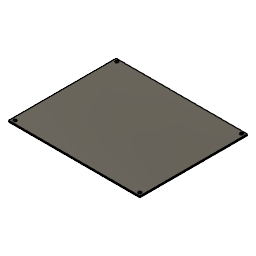
BB-BOT (Autodesk Fusion 360 archive; units mm, degrees)
design "Top plate"
Autodesk Fusion 360 part; units mm, degrees
sketch "Sketch1" plane through (0, 0, 45) normal (0, 0, 1) x (-1, 0, 0) in component "Top guard"
  arc A0 (130, -95) -> (130, -75) centre (130, -85) ccw
  line L0 (130, -75) -> (120, -75)
  line L1 (120, -75) -> (120, -35)
  line L2 (120, -35) -> (130, -35)
  arc A1 (130, -35) -> (130, -15) centre (130, -25) ccw
  line L3 (130, -15) -> (100, -15)
  line L4 (100, -15) -> (100, 50)
  line L5 (100, 50) -> (-100, 50)
  line L6 (-100, 50) -> (-100, -15)
  line L7 (-100, -15) -> (-130, -15)
  arc A2 (-130, -15) -> (-130, -35) centre (-130, -25) ccw
  line L8 (-130, -35) -> (-120, -35)
  line L9 (-120, -35) -> (-120, -75)
  line L10 (-120, -75) -> (-129.9999, -75)
  arc A3 (-129.9999, -75) -> (-129.9999, -95) centre (-129.9999, -85) ccw
  line L11 (-129.9999, -95) -> (-100, -95)
  line L12 (-100, -95) -> (-100, -160)
  line L13 (-100, -160) -> (-74, -160)
  line L14 (-74, -160) -> (-74, -115)
  line L15 (-74, -115) -> (74, -115)
  line L16 (74, -115) -> (74, -160)
  line L17 (74, -160) -> (100, -160)
  line L18 (100, -160) -> (100, -95)
  line L19 (100, -95) -> (130, -95)
  line L20 (83, 45) -> (83, -109)
  line L21 (-83, -109) -> (-83, 45)
  line L22 (-83, 45) -> (83, 45)
  circle A4 centre (130, -25) radius 4
  circle A5 centre (-129.9999, -85) radius 4
  circle A6 centre (-130, -25) radius 4
  circle A7 centre (130, -85) radius 4
  line L23 (100, -114) -> (-100, -114)
  line L24 (-100, -114) -> (-100, 50)
  line L25 (-100, 50) -> (100, 50)
  line L26 (100, 50) -> (100, -114)
  circle A8 centre (-95, -110) radius 2.25
  circle A9 centre (95, -110) radius 2.25
  circle A10 centre (95, 45) radius 2.25
  circle A11 centre (-95, 45) radius 2.25
  dimension "d7" = 4.5
  dimension "d8" = 4.5
  dimension "d9" = 4.5
  dimension "d10" = 4.5
  constraint horizontal L23
  constraint vertical L24
  constraint horizontal L25
  constraint vertical L26
  constraint coincident L5.end L6.start
  constraint coincident L18 L23.start
  measures "d7" diameter of A8
  measures "d8" diameter of A9
  measures "d9" diameter of A10
  measures "d10" diameter of A11
extrude "Extrude1" add sketch "Sketch1" along normal blind 2 contours L4 L5 L6 L12 L18 L23 L24 L25 L26 | A8 | A9 | A10 | A11 in component "Top guard"
extrude "Extrude2" cut sketch "Sketch1" along normal blind 2 contours A8 | A9 | A10 | A11 in component "Top guard"
component "Top guard" placed x (1, 0, 0) y (0, 1, 0) z (0, 0, 1) at (0, 0, 0)

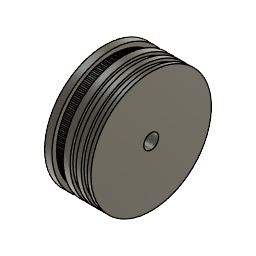
design "Wheel Hub"
Autodesk Fusion 360 part; units mm, degrees
sketch "Sketch1" plane through (0, 0, 0) normal (1, 0, 0) x (0, 1, 0) in component "Wheel-Hub"
  circle A0 centre (0, 0) radius 32.5
  dimension "d1" = 65
  constraint coincident A0.centre origin
  measures "d1" diameter of A0
extrude "Extrude1" add sketch "Sketch1" along normal blind 25 in component "Wheel-Hub"
sketch "Sketch2" plane through (25, 0, 0) normal (1, 0, 0) x (0, 1, 0) in component "Wheel-Hub"
  circle A0 centre (0, 0) radius 32.5
  circle A1 centre (0, 0) radius 4
  constraint coincident A0.centre A1.centre
extrude "Extrude2" cut sketch "Sketch2" against normal blind 25 contours A1 in component "Wheel-Hub"
sketch "Sketch3" plane through (25, 0, 0) normal (1, 0, 0) x (0, 1, 0) in component "Wheel-Hub"
  circle A0 centre (0, 0) radius 4
  circle A1 centre (0, 0) radius 32.5
  circle A2 centre (0, 0) radius 32.5
  circle A3 centre (0, 0) radius 31
  dimension "d6" = 65
  dimension "d7" = 62
  constraint coincident A0.centre A1.centre
  constraint concentric A2 A3
  measures "d6" diameter of A2
  measures "d7" diameter of A3
extrude "Extrude3" cut sketch "Sketch3" against normal blind 3.2 from surface at -2 contours A1 A2 in component "Wheel-Hub"
extrude "Extrude4" cut sketch "Sketch3" against normal blind 3.2 from surface at -8 contours A1 A2 in component "Wheel-Hub"
sketch "Sketch4" plane through (25, 0, 0) normal (1, 0, 0) x (0, 1, 0) in component "Wheel-Hub"
  circle A0 centre (0, 0) radius 4
  circle A1 centre (0, 0) radius 32.5
  circle A2 centre (0, 0) radius 32.5
  circle A3 centre (0, 0) radius 30
  dimension "d14" = 65
  dimension "d15" = 60
  constraint coincident A0.centre A1.centre
  measures "d14" diameter of A2
  measures "d15" diameter of A3
extrude "Extrude5" cut sketch "Sketch4" against normal blind 6 from surface at -15 contours A1 A2 in component "Wheel-Hub"
sketch "Sketch1 (2)" plane through (4, 0, 0) normal (1, 0, 0) x (0, 1, 0)
  circle A0 centre (0, 0) radius 30
  circle A1 centre (0, 0) radius 32.5
  line L0 (30, 0) -> (20.725, 0)
  line L1 (30, 0) -> (29.3, 0)
  line L2 (29.3, 0.5) -> (29.3, -0.5)
  line L3 (29.3, 0.5) -> (29.97, 0.7439)
  line L4 (29.3, -0.5) -> (29.97, -0.7439)
  arc A2 (29.97, -0.7439) -> (29.97, 0.7439) centre (20.7626, 0) ccw
  line L5 (29.3, 0) -> (29.315, 0)
  arc A3 (29.3, -0.5) -> (29.3, 0.5) centre (20.9742, 0) ccw
  line L6 (29.1677, 2.8263) -> (29.8162, 3.1226)
  arc A4 (29.9344, 1.6396) -> (29.8162, 3.1226) centre (20.697, 1.6496) ccw
  line L7 (29.2471, 1.8295) -> (29.9344, 1.6396)
  arc A5 (29.2471, 1.8295) -> (29.1677, 2.8263) centre (20.9079, 1.6664) ccw
  line L8 (28.8509, 5.1347) -> (29.4738, 5.4817)
  arc A6 (29.7095, 4.0127) -> (29.4738, 5.4817) centre (20.5005, 3.2888) ccw
  line L9 (29.0093, 4.1474) -> (29.7095, 4.0127)
  arc A7 (29.0093, 4.1474) -> (28.8509, 5.1347) centre (20.7094, 3.3223) ccw
  line L10 (28.3517, 7.4107) -> (28.9451, 7.806)
  arc A8 (29.2967, 6.3605) -> (28.9451, 7.806) centre (20.1744, 4.9071) ccw
  line L11 (28.5881, 6.4391) -> (29.2967, 6.3605)
  arc A9 (28.5881, 6.4391) -> (28.3517, 7.4107) centre (20.3799, 4.9571) ccw
  line L12 (27.6733, 9.6399) -> (28.2334, 10.081)
  arc A10 (28.6988, 8.668) -> (28.2334, 10.081) centre (19.7207, 6.4945) ccw
  line L13 (27.9861, 8.69) -> (28.6988, 8.668)
  arc A11 (27.9861, 8.69) -> (27.6733, 9.6399) centre (19.9217, 6.5606) ccw
  line L14 (26.82, 11.808) -> (27.3432, 12.2923)
  arc A12 (27.9194, 10.9207) -> (27.3432, 12.2923) centre (19.1424, 8.0408) ccw
  line L15 (27.2072, 10.8861) -> (27.9194, 10.9207)
  arc A13 (27.2072, 10.8861) -> (26.82, 11.808) centre (19.3375, 8.1227) ccw
  line L16 (25.797, 13.9016) -> (26.2802, 14.4259)
  arc A14 (26.9635, 13.1044) -> (26.2802, 14.4259) centre (18.4431, 9.5362) ccw
  line L17 (26.2563, 13.0133) -> (26.9635, 13.1044)
  arc A15 (26.2563, 13.0133) -> (25.797, 13.9016) centre (18.631, 9.6334) ccw
  line L18 (24.611, 15.9072) -> (25.051, 16.4683)
  arc A16 (25.8371, 15.2052) -> (25.051, 16.4683) centre (17.6271, 10.9714) ccw
  line L19 (25.1394, 15.0582) -> (25.8371, 15.2052)
  arc A17 (25.1394, 15.0582) -> (24.611, 15.9072) centre (17.8067, 11.0832) ccw
  line L20 (23.2694, 17.8122) -> (23.6634, 18.4065)
  arc A18 (24.5474, 17.2099) -> (23.6634, 18.4065) centre (16.6997, 12.3372) ccw
  line L21 (23.8636, 17.0079) -> (24.5474, 17.2099)
  arc A19 (23.8636, 17.0079) -> (23.2694, 17.8122) centre (16.8699, 12.4629) ccw
  line L22 (21.7806, 19.6047) -> (22.1262, 20.2284)
  arc A20 (23.1024, 19.1058) -> (22.1262, 20.2284) centre (15.6667, 13.625) ccw
  line L23 (22.4369, 18.8501) -> (23.1024, 19.1058)
  arc A21 (22.4369, 18.8501) -> (21.7806, 19.6047) centre (15.8264, 13.7638) ccw
  line L24 (20.1542, 21.2732) -> (20.4491, 21.9224)
  arc A22 (21.5115, 20.8809) -> (20.4491, 21.9224) centre (14.5347, 14.8266) ccw
  line L25 (20.8683, 20.5732) -> (21.5115, 20.8809)
  arc A23 (20.8683, 20.5732) -> (20.1542, 21.2732) centre (14.6828, 14.9777) ccw
  line L26 (18.4003, 22.8072) -> (18.6427, 23.4777)
  arc A24 (19.7845, 22.524) -> (18.6427, 23.4777) centre (13.3108, 15.9345) ccw
  line L27 (19.1678, 22.1661) -> (19.7845, 22.524)
  arc A25 (19.1678, 22.1661) -> (18.4003, 22.8072) centre (13.4464, 16.0969) ccw
  line L28 (16.5301, 24.197) -> (16.7184, 24.8847)
  arc A26 (17.9324, 24.0246) -> (16.7184, 24.8847) centre (12.0027, 16.9417) ccw
  line L29 (17.3461, 23.6189) -> (17.9324, 24.0246)
  arc A27 (17.3461, 23.6189) -> (16.5301, 24.197) centre (12.125, 17.1143) ccw
  line L30 (14.5554, 25.4338) -> (14.6885, 26.1343)
  arc A28 (15.9669, 25.3734) -> (14.6885, 26.1343) centre (10.6187, 17.8418) ccw
  line L31 (15.4147, 24.9224) -> (15.9669, 25.3734)
  arc A29 (15.4147, 24.9224) -> (14.5554, 25.4338) centre (10.7269, 18.0235) ccw
  line L32 (12.4887, 26.5099) -> (12.5657, 27.2187)
  arc A30 (13.9005, 26.5618) -> (12.5657, 27.2187) centre (9.1676, 18.629) ccw
  line L33 (13.3859, 26.0683) -> (13.9005, 26.5618)
  arc A31 (13.3859, 26.0683) -> (12.4887, 26.5099) centre (9.261, 18.8188) ccw
  line L34 (10.343, 27.4183) -> (10.3634, 28.131)
  arc A32 (11.7463, 27.5822) -> (10.3634, 28.131) centre (7.6586, 19.2985) ccw
  line L35 (11.2725, 27.0494) -> (11.7463, 27.5822)
  arc A33 (11.2725, 27.0494) -> (10.343, 27.4183) centre (7.7366, 19.4951) ccw
  line L36 (8.1319, 28.1534) -> (8.0957, 28.8655)
  arc A34 (9.5177, 28.4283) -> (8.0957, 28.8655) centre (6.1011, 19.846) ccw
  line L37 (9.0877, 27.8595) -> (9.5177, 28.4283)
  arc A35 (9.0877, 27.8595) -> (8.1319, 28.1534) centre (6.1633, 20.0482) ccw
  line L38 (5.8694, 28.7105) -> (5.7767, 29.4174)
  arc A36 (7.229, 29.0946) -> (5.7767, 29.4174) centre (4.505, 20.268) ccw
  line L39 (6.8456, 28.4935) -> (7.229, 29.0946)
  arc A37 (6.8456, 28.4935) -> (5.8694, 28.7105) centre (4.5509, 20.4745) ccw
  line L40 (3.5698, 29.086) -> (3.4212, 29.7834)
  arc A38 (4.8946, 29.577) -> (3.4212, 29.7834) centre (2.8805, 20.5618) ccw
  line L41 (4.5601, 28.9473) -> (4.8946, 29.577)
  arc A39 (4.5601, 28.9473) -> (3.5698, 29.086) centre (2.9099, 20.7713) ccw
  line L42 (1.2476, 29.2777) -> (1.0441, 29.961)
  arc A40 (2.5292, 29.8724) -> (1.0441, 29.961) centre (1.2378, 20.7257) ccw
  line L43 (2.2458, 29.2181) -> (2.5292, 29.8724)
  arc A41 (2.2458, 29.2181) -> (1.2476, 29.2777) centre (1.2504, 20.9369) ccw
  line L44 (-1.0824, 29.2843) -> (-1.3396, 29.9493)
  arc A42 (0.1478, 29.9789) -> (-1.3396, 29.9493) centre (-0.4128, 20.7585) ccw
  line L45 (-0.0826, 29.3041) -> (0.1478, 29.9789)
  arc A43 (-0.0826, 29.3041) -> (-1.0824, 29.2843) centre (-0.417, 20.97) ccw
  line L46 (-3.4057, 29.1057) -> (-3.7148, 29.7482)
  arc A44 (-2.2344, 29.8958) -> (-3.7148, 29.7482) centre (-2.0608, 20.6601) ccw
  line L47 (-2.4106, 29.2049) -> (-2.2344, 29.8958)
  arc A45 (-2.4106, 29.2049) -> (-3.4057, 29.1057) centre (-2.0818, 20.8706) ccw
  line L48 (-5.7074, 28.7431) -> (-6.0666, 29.359)
  arc A46 (-4.6026, 29.6238) -> (-6.0666, 29.359) centre (-3.6957, 20.431) ccw
  line L49 (-4.7233, 28.9211) -> (-4.6026, 29.6238)
  arc A47 (-4.7233, 28.9211) -> (-5.7074, 28.7431) centre (-3.7334, 20.6392) ccw
  line L50 (-7.973, 28.1988) -> (-8.38, 28.7842)
  arc A48 (-6.9417, 29.1645) -> (-8.38, 28.7842) centre (-5.3073, 20.0728) ccw
  line L51 (-7.0062, 28.4544) -> (-6.9417, 29.1645)
  arc A49 (-7.0062, 28.4544) -> (-7.973, 28.1988) centre (-5.3613, 20.2774) ccw
  line L52 (-10.1882, 27.4762) -> (-10.6404, 28.0274)
  arc A50 (-9.2369, 28.5208) -> (-10.6404, 28.0274) centre (-6.8853, 19.5877) ccw
  line L53 (-9.2447, 27.8078) -> (-9.2369, 28.5208)
  arc A51 (-9.2447, 27.8078) -> (-10.1882, 27.4762) centre (-6.9554, 19.7873) ccw
  line L54 (-12.3389, 26.5799) -> (-12.8335, 27.0934)
  arc A52 (-11.4736, 27.6967) -> (-12.8335, 27.0934) centre (-8.4198, 18.9788) ccw
  line L55 (-11.4248, 26.9854) -> (-11.4736, 27.6967)
  arc A53 (-11.4248, 26.9854) -> (-12.3389, 26.5799) centre (-8.5056, 19.1721) ccw
  line L56 (-14.4117, 25.5155) -> (-14.9456, 25.9882)
  arc A54 (-13.6379, 26.6976) -> (-14.9456, 25.9882) centre (-9.901, 18.2498) ccw
  line L57 (-13.5327, 25.9924) -> (-13.6379, 26.6976)
  arc A55 (-13.5327, 25.9924) -> (-14.4117, 25.5155) centre (-10.0019, 18.4358) ccw
  line L58 (-16.3934, 24.2899) -> (-16.9631, 24.7186)
  arc A56 (-15.7159, 25.5297) -> (-16.9631, 24.7186) centre (-11.3197, 17.4055) ccw
  line L59 (-15.5551, 24.8351) -> (-15.7159, 25.5297)
  arc A57 (-15.5551, 24.8351) -> (-16.3934, 24.2899) centre (-11.435, 17.5828) ccw
  line L60 (-18.2714, 22.9106) -> (-18.8733, 23.2927)
  arc A58 (-17.6946, 24.2003) -> (-18.8733, 23.2927) centre (-12.6667, 16.4511) ccw
  line L61 (-17.479, 23.5207) -> (-17.6946, 24.2003)
  arc A59 (-17.479, 23.5207) -> (-18.2714, 22.9106) centre (-12.7958, 16.6187) ccw
  line L62 (-20.0339, 21.3865) -> (-20.6643, 21.7196)
  arc A60 (-19.5613, 22.718) -> (-20.6643, 21.7196) centre (-13.9337, 15.3927) ccw
  line L63 (-19.2925, 22.0576) -> (-19.5613, 22.718)
  arc A61 (-19.2925, 22.0576) -> (-20.0339, 21.3865) centre (-14.0757, 15.5496) ccw
  line L64 (-21.6697, 19.7272) -> (-22.3246, 20.0092)
  arc A62 (-21.3045, 21.092) -> (-22.3246, 20.0092) centre (-15.1127, 14.237) ccw
  line L65 (-20.984, 20.4551) -> (-21.3045, 21.092)
  arc A63 (-20.984, 20.4551) -> (-21.6697, 19.7272) centre (-15.2666, 14.3821) ccw
  line L66 (-23.1685, 17.9432) -> (-23.8438, 18.1722)
  arc A64 (-22.9129, 19.3327) -> (-23.8438, 18.1722) centre (-16.196, 12.9913) ccw
  line L67 (-22.5428, 18.7233) -> (-22.9129, 19.3327)
  arc A65 (-22.5428, 18.7233) -> (-23.1685, 17.9432) centre (-16.361, 13.1237) ccw
  line L68 (-24.5209, 16.0458) -> (-25.2122, 16.2204)
  arc A66 (-24.3764, 17.4512) -> (-25.2122, 16.2204) centre (-17.177, 11.6635) ccw
  line L69 (-23.9591, 16.8731) -> (-24.3764, 17.4512)
  arc A67 (-23.9591, 16.8731) -> (-24.5209, 16.0458) centre (-17.352, 11.7823) ccw
  line L70 (-25.7182, 14.0468) -> (-26.4212, 14.166)
  arc A68 (-25.6859, 15.4593) -> (-26.4212, 14.166) centre (-18.0493, 10.2619) ccw
  line L71 (-25.224, 14.9162) -> (-25.6859, 15.4593)
  arc A69 (-25.224, 14.9162) -> (-25.7182, 14.0468) centre (-18.2333, 10.3665) ccw
  line L72 (-26.7529, 11.9591) -> (-27.4632, 12.022)
  arc A70 (-26.8329, 13.3697) -> (-27.4632, 12.022) centre (-18.8076, 8.7954) ccw
  line L73 (-26.3293, 12.865) -> (-26.8329, 13.3697)
  arc A71 (-26.3293, 12.865) -> (-26.7529, 11.9591) centre (-18.9992, 8.8851) ccw
  line L74 (-27.6185, 9.7958) -> (-28.3315, 9.8021)
  arc A72 (-27.8103, 11.1955) -> (-28.3315, 9.8021) centre (-19.4469, 7.2734) ccw
  line L75 (-27.2682, 10.7324) -> (-27.8103, 11.1955)
  arc A73 (-27.2682, 10.7324) -> (-27.6185, 9.7958) centre (-19.6451, 7.3475) ccw
  line L76 (-28.3095, 7.5705) -> (-29.0207, 7.5202)
  arc A74 (-28.6119, 8.9506) -> (-29.0207, 7.5202) centre (-19.9633, 5.7053) ccw
  line L77 (-28.0347, 8.532) -> (-28.6119, 8.9506)
  arc A75 (-28.0347, 8.532) -> (-28.3095, 7.5705) centre (-20.1668, 5.7634) ccw
  line L78 (-28.8215, 5.2974) -> (-29.5264, 5.1907)
  arc A76 (-29.2326, 6.6491) -> (-29.5264, 5.1907) centre (-20.3535, 4.1012) ccw
  line L79 (-28.6239, 6.2777) -> (-29.2326, 6.6491)
  arc A77 (-28.6239, 6.2777) -> (-28.8215, 5.2974) centre (-20.5609, 4.143) ccw
  line L80 (-29.1512, 2.9908) -> (-29.8455, 2.8284)
  arc A78 (-29.6684, 4.3055) -> (-29.8455, 2.8284) centre (-20.615, 2.4711) ccw
  line L81 (-29.0322, 3.9837) -> (-29.6684, 4.3055)
  arc A79 (-29.0322, 3.9837) -> (-29.1512, 2.9908) centre (-20.8251, 2.4963) ccw
  line L82 (-29.2967, 0.6653) -> (-29.9759, 0.4482)
  arc A80 (-29.9167, 1.9348) -> (-29.9759, 0.4482) centre (-20.7462, 0.8254) ccw
  line L83 (-29.257, 1.6645) -> (-29.9167, 1.9348)
  arc A81 (-29.257, 1.6645) -> (-29.2967, 0.6653) centre (-20.9576, 0.8339) ccw
  line L84 (-29.257, -1.6645) -> (-29.9167, -1.9348)
  arc A82 (-29.9759, -0.4482) -> (-29.9167, -1.9348) centre (-20.7462, -0.8254) ccw
  line L85 (-29.2967, -0.6653) -> (-29.9759, -0.4482)
  arc A83 (-29.2967, -0.6653) -> (-29.257, -1.6645) centre (-20.9576, -0.8339) ccw
  line L86 (-29.0322, -3.9837) -> (-29.6684, -4.3055)
  arc A84 (-29.8455, -2.8284) -> (-29.6684, -4.3055) centre (-20.615, -2.4711) ccw
  line L87 (-29.1512, -2.9908) -> (-29.8455, -2.8284)
  arc A85 (-29.1512, -2.9908) -> (-29.0322, -3.9837) centre (-20.8251, -2.4963) ccw
  line L88 (-28.6239, -6.2777) -> (-29.2326, -6.6491)
  arc A86 (-29.5264, -5.1907) -> (-29.2326, -6.6491) centre (-20.3535, -4.1012) ccw
  line L89 (-28.8215, -5.2974) -> (-29.5264, -5.1907)
  arc A87 (-28.8215, -5.2974) -> (-28.6239, -6.2777) centre (-20.5609, -4.143) ccw
  line L90 (-28.0347, -8.532) -> (-28.6119, -8.9506)
  arc A88 (-29.0207, -7.5202) -> (-28.6119, -8.9506) centre (-19.9633, -5.7053) ccw
  line L91 (-28.3095, -7.5705) -> (-29.0207, -7.5202)
  arc A89 (-28.3095, -7.5705) -> (-28.0347, -8.532) centre (-20.1668, -5.7634) ccw
  line L92 (-27.2682, -10.7324) -> (-27.8103, -11.1955)
  arc A90 (-28.3315, -9.8021) -> (-27.8103, -11.1955) centre (-19.4469, -7.2734) ccw
  line L93 (-27.6185, -9.7958) -> (-28.3315, -9.8021)
  arc A91 (-27.6185, -9.7958) -> (-27.2682, -10.7324) centre (-19.6451, -7.3475) ccw
  line L94 (-26.3293, -12.865) -> (-26.8329, -13.3697)
  arc A92 (-27.4632, -12.022) -> (-26.8329, -13.3697) centre (-18.8076, -8.7954) ccw
  line L95 (-26.7529, -11.9591) -> (-27.4632, -12.022)
  arc A93 (-26.7529, -11.9591) -> (-26.3293, -12.865) centre (-18.9992, -8.8851) ccw
  line L96 (-25.224, -14.9162) -> (-25.6859, -15.4593)
  arc A94 (-26.4212, -14.166) -> (-25.6859, -15.4593) centre (-18.0493, -10.2619) ccw
  line L97 (-25.7182, -14.0468) -> (-26.4212, -14.166)
  arc A95 (-25.7182, -14.0468) -> (-25.224, -14.9162) centre (-18.2333, -10.3665) ccw
  line L98 (-23.9591, -16.8731) -> (-24.3764, -17.4512)
  arc A96 (-25.2122, -16.2204) -> (-24.3764, -17.4512) centre (-17.177, -11.6635) ccw
  line L99 (-24.5209, -16.0458) -> (-25.2122, -16.2204)
  arc A97 (-24.5209, -16.0458) -> (-23.9591, -16.8731) centre (-17.352, -11.7823) ccw
  line L100 (-22.5428, -18.7233) -> (-22.9129, -19.3327)
  arc A98 (-23.8438, -18.1722) -> (-22.9129, -19.3327) centre (-16.196, -12.9913) ccw
  line L101 (-23.1685, -17.9432) -> (-23.8438, -18.1722)
  arc A99 (-23.1685, -17.9432) -> (-22.5428, -18.7233) centre (-16.361, -13.1237) ccw
  line L102 (-20.984, -20.4551) -> (-21.3045, -21.092)
  arc A100 (-22.3246, -20.0092) -> (-21.3045, -21.092) centre (-15.1127, -14.237) ccw
  line L103 (-21.6697, -19.7272) -> (-22.3246, -20.0092)
  arc A101 (-21.6697, -19.7272) -> (-20.984, -20.4551) centre (-15.2666, -14.3821) ccw
  line L104 (-19.2925, -22.0576) -> (-19.5613, -22.718)
  arc A102 (-20.6643, -21.7196) -> (-19.5613, -22.718) centre (-13.9337, -15.3927) ccw
  line L105 (-20.0339, -21.3865) -> (-20.6643, -21.7196)
  arc A103 (-20.0339, -21.3865) -> (-19.2925, -22.0576) centre (-14.0757, -15.5496) ccw
  line L106 (-17.479, -23.5207) -> (-17.6946, -24.2003)
  arc A104 (-18.8733, -23.2927) -> (-17.6946, -24.2003) centre (-12.6667, -16.4511) ccw
  line L107 (-18.2714, -22.9106) -> (-18.8733, -23.2927)
  arc A105 (-18.2714, -22.9106) -> (-17.479, -23.5207) centre (-12.7958, -16.6187) ccw
  line L108 (-15.5551, -24.8351) -> (-15.7159, -25.5297)
  arc A106 (-16.9631, -24.7186) -> (-15.7159, -25.5297) centre (-11.3197, -17.4055) ccw
  line L109 (-16.3934, -24.2899) -> (-16.9631, -24.7186)
  arc A107 (-16.3934, -24.2899) -> (-15.5551, -24.8351) centre (-11.435, -17.5828) ccw
  line L110 (-13.5327, -25.9924) -> (-13.6379, -26.6976)
  arc A108 (-14.9456, -25.9882) -> (-13.6379, -26.6976) centre (-9.901, -18.2498) ccw
  line L111 (-14.4117, -25.5155) -> (-14.9456, -25.9882)
  arc A109 (-14.4117, -25.5155) -> (-13.5327, -25.9924) centre (-10.0019, -18.4358) ccw
  line L112 (-11.4248, -26.9854) -> (-11.4736, -27.6967)
  arc A110 (-12.8335, -27.0934) -> (-11.4736, -27.6967) centre (-8.4198, -18.9788) ccw
  line L113 (-12.3389, -26.5799) -> (-12.8335, -27.0934)
  arc A111 (-12.3389, -26.5799) -> (-11.4248, -26.9854) centre (-8.5056, -19.1721) ccw
  line L114 (-9.2447, -27.8078) -> (-9.2369, -28.5208)
  arc A112 (-10.6404, -28.0274) -> (-9.2369, -28.5208) centre (-6.8853, -19.5877) ccw
  line L115 (-10.1882, -27.4762) -> (-10.6404, -28.0274)
  arc A113 (-10.1882, -27.4762) -> (-9.2447, -27.8078) centre (-6.9554, -19.7873) ccw
  line L116 (-7.0062, -28.4544) -> (-6.9417, -29.1645)
  arc A114 (-8.38, -28.7842) -> (-6.9417, -29.1645) centre (-5.3073, -20.0728) ccw
  line L117 (-7.973, -28.1988) -> (-8.38, -28.7842)
  arc A115 (-7.973, -28.1988) -> (-7.0062, -28.4544) centre (-5.3613, -20.2774) ccw
  line L118 (-4.7233, -28.9211) -> (-4.6026, -29.6238)
  arc A116 (-6.0666, -29.359) -> (-4.6026, -29.6238) centre (-3.6957, -20.431) ccw
  line L119 (-5.7074, -28.7431) -> (-6.0666, -29.359)
  arc A117 (-5.7074, -28.7431) -> (-4.7233, -28.9211) centre (-3.7334, -20.6392) ccw
  line L120 (-2.4106, -29.2049) -> (-2.2344, -29.8958)
  arc A118 (-3.7148, -29.7482) -> (-2.2344, -29.8958) centre (-2.0608, -20.6601) ccw
  line L121 (-3.4057, -29.1057) -> (-3.7148, -29.7482)
  arc A119 (-3.4057, -29.1057) -> (-2.4106, -29.2049) centre (-2.0818, -20.8706) ccw
  line L122 (-0.0826, -29.3041) -> (0.1478, -29.9789)
  arc A120 (-1.3396, -29.9493) -> (0.1478, -29.9789) centre (-0.4128, -20.7585) ccw
  line L123 (-1.0824, -29.2843) -> (-1.3396, -29.9493)
  arc A121 (-1.0824, -29.2843) -> (-0.0826, -29.3041) centre (-0.417, -20.97) ccw
  line L124 (2.2458, -29.2181) -> (2.5292, -29.8724)
  arc A122 (1.0441, -29.961) -> (2.5292, -29.8724) centre (1.2378, -20.7257) ccw
  line L125 (1.2476, -29.2777) -> (1.0441, -29.961)
  arc A123 (1.2476, -29.2777) -> (2.2458, -29.2181) centre (1.2504, -20.9369) ccw
  line L126 (4.5601, -28.9473) -> (4.8946, -29.577)
  arc A124 (3.4212, -29.7834) -> (4.8946, -29.577) centre (2.8805, -20.5618) ccw
  line L127 (3.5698, -29.086) -> (3.4212, -29.7834)
  arc A125 (3.5698, -29.086) -> (4.5601, -28.9473) centre (2.9099, -20.7713) ccw
  line L128 (6.8456, -28.4935) -> (7.229, -29.0946)
  arc A126 (5.7767, -29.4174) -> (7.229, -29.0946) centre (4.505, -20.268) ccw
  line L129 (5.8694, -28.7105) -> (5.7767, -29.4174)
  arc A127 (5.8694, -28.7105) -> (6.8456, -28.4935) centre (4.5509, -20.4745) ccw
  line L130 (9.0877, -27.8595) -> (9.5177, -28.4283)
  arc A128 (8.0957, -28.8655) -> (9.5177, -28.4283) centre (6.1011, -19.846) ccw
  line L131 (8.1319, -28.1534) -> (8.0957, -28.8655)
  arc A129 (8.1319, -28.1534) -> (9.0877, -27.8595) centre (6.1633, -20.0482) ccw
  line L132 (11.2725, -27.0494) -> (11.7463, -27.5822)
  arc A130 (10.3634, -28.131) -> (11.7463, -27.5822) centre (7.6586, -19.2985) ccw
  line L133 (10.343, -27.4183) -> (10.3634, -28.131)
  arc A131 (10.343, -27.4183) -> (11.2725, -27.0494) centre (7.7366, -19.4951) ccw
  line L134 (13.3859, -26.0683) -> (13.9005, -26.5618)
  arc A132 (12.5657, -27.2187) -> (13.9005, -26.5618) centre (9.1676, -18.629) ccw
  line L135 (12.4887, -26.5099) -> (12.5657, -27.2187)
  arc A133 (12.4887, -26.5099) -> (13.3859, -26.0683) centre (9.261, -18.8188) ccw
  line L136 (15.4147, -24.9224) -> (15.9669, -25.3734)
  arc A134 (14.6885, -26.1343) -> (15.9669, -25.3734) centre (10.6187, -17.8418) ccw
  line L137 (14.5554, -25.4338) -> (14.6885, -26.1343)
  arc A135 (14.5554, -25.4338) -> (15.4147, -24.9224) centre (10.7269, -18.0235) ccw
  line L138 (17.3461, -23.6189) -> (17.9324, -24.0246)
  arc A136 (16.7184, -24.8847) -> (17.9324, -24.0246) centre (12.0027, -16.9417) ccw
  line L139 (16.5301, -24.197) -> (16.7184, -24.8847)
  arc A137 (16.5301, -24.197) -> (17.3461, -23.6189) centre (12.125, -17.1143) ccw
  line L140 (19.1678, -22.1661) -> (19.7845, -22.524)
  arc A138 (18.6427, -23.4777) -> (19.7845, -22.524) centre (13.3108, -15.9345) ccw
  line L141 (18.4003, -22.8072) -> (18.6427, -23.4777)
  arc A139 (18.4003, -22.8072) -> (19.1678, -22.1661) centre (13.4464, -16.0969) ccw
  line L142 (20.8683, -20.5732) -> (21.5115, -20.8809)
  arc A140 (20.4491, -21.9224) -> (21.5115, -20.8809) centre (14.5347, -14.8266) ccw
  line L143 (20.1542, -21.2732) -> (20.4491, -21.9224)
  arc A141 (20.1542, -21.2732) -> (20.8683, -20.5732) centre (14.6828, -14.9777) ccw
  line L144 (22.4369, -18.8501) -> (23.1024, -19.1058)
  arc A142 (22.1262, -20.2284) -> (23.1024, -19.1058) centre (15.6667, -13.625) ccw
  line L145 (21.7806, -19.6047) -> (22.1262, -20.2284)
  arc A143 (21.7806, -19.6047) -> (22.4369, -18.8501) centre (15.8264, -13.7638) ccw
  line L146 (23.8636, -17.0079) -> (24.5474, -17.2099)
  arc A144 (23.6634, -18.4065) -> (24.5474, -17.2099) centre (16.6997, -12.3372) ccw
  line L147 (23.2694, -17.8122) -> (23.6634, -18.4065)
  arc A145 (23.2694, -17.8122) -> (23.8636, -17.0079) centre (16.8699, -12.4629) ccw
  line L148 (25.1394, -15.0582) -> (25.8371, -15.2052)
  arc A146 (25.051, -16.4683) -> (25.8371, -15.2052) centre (17.6271, -10.9714) ccw
  line L149 (24.611, -15.9072) -> (25.051, -16.4683)
  arc A147 (24.611, -15.9072) -> (25.1394, -15.0582) centre (17.8067, -11.0832) ccw
  line L150 (26.2563, -13.0133) -> (26.9635, -13.1044)
  arc A148 (26.2802, -14.4259) -> (26.9635, -13.1044) centre (18.4431, -9.5362) ccw
  line L151 (25.797, -13.9016) -> (26.2802, -14.4259)
  arc A149 (25.797, -13.9016) -> (26.2563, -13.0133) centre (18.631, -9.6334) ccw
  line L152 (27.2072, -10.8861) -> (27.9194, -10.9207)
  arc A150 (27.3432, -12.2923) -> (27.9194, -10.9207) centre (19.1424, -8.0408) ccw
  line L153 (26.82, -11.808) -> (27.3432, -12.2923)
  arc A151 (26.82, -11.808) -> (27.2072, -10.8861) centre (19.3375, -8.1227) ccw
  line L154 (27.9861, -8.69) -> (28.6988, -8.668)
  arc A152 (28.2334, -10.081) -> (28.6988, -8.668) centre (19.7207, -6.4945) ccw
  line L155 (27.6733, -9.6399) -> (28.2334, -10.081)
  arc A153 (27.6733, -9.6399) -> (27.9861, -8.69) centre (19.9217, -6.5606) ccw
  line L156 (28.5881, -6.4391) -> (29.2967, -6.3605)
  arc A154 (28.9451, -7.806) -> (29.2967, -6.3605) centre (20.1744, -4.9071) ccw
  line L157 (28.3517, -7.4107) -> (28.9451, -7.806)
  arc A155 (28.3517, -7.4107) -> (28.5881, -6.4391) centre (20.3799, -4.9571) ccw
  line L158 (29.0093, -4.1474) -> (29.7095, -4.0127)
  arc A156 (29.4738, -5.4817) -> (29.7095, -4.0127) centre (20.5005, -3.2888) ccw
  line L159 (28.8509, -5.1347) -> (29.4738, -5.4817)
  arc A157 (28.8509, -5.1347) -> (29.0093, -4.1474) centre (20.7094, -3.3223) ccw
  line L160 (29.2471, -1.8295) -> (29.9344, -1.6396)
  arc A158 (29.8162, -3.1226) -> (29.9344, -1.6396) centre (20.697, -1.6496) ccw
  line L161 (29.1677, -2.8263) -> (29.8162, -3.1226)
  arc A159 (29.1677, -2.8263) -> (29.2471, -1.8295) centre (20.9079, -1.6664) ccw
  dimension "d19" = 9.275
  dimension "d20" = 0.7
  dimension "d21" = 1
  dimension "d22" = 0.713
  dimension "d23" = 0.713
  dimension "d24" = 110
  dimension "d25" = 110
  dimension "d26" = 0.015
  dimension "d28" = 360
  constraint coincident A0 L0.start
  constraint horizontal L0
  constraint parallel L0 L1
  constraint perpendicular L0 L2
  constraint coincident L0.start A2
  constraint perpendicular L2 L5
  constraint coincident L5.end A3
  measures "d19" distance of L0.start L0.end
  measures "d20" distance of L0.start L1.end
  measures "d21" distance of L2.start L2.end
  measures "d22" distance of L2.start L3.end
  measures "d23" distance of L2.end L4.end
  measures "d24" angle of L2 L3
  measures "d25" angle of L2 L4
  measures "d26" distance of L1.end L5.end
extrude "Extrude6" cut sketch "Sketch1 (2)" along normal blind 6 contours L6 A4 L7 A5 | L8 A6 L9 A7 | L10 A8 L11 A9 | L12 A10 L13 A11 | L14 A12 L15 A13 | L16 A14 L17 A15 | L18 A16 L19 A17 | L20 A18 L21 A19 | L22 A20 L23 A21 | L24 A22 L25 A23 | L26 A24 L27 A25 | L28 A26 L29 A27 | L30 A28 L31 A29 | L32 A30 L33 A31 | L34 A32 L35 A33 | L36 A34 L37 A35 | L38 A36 L39 A37 | L40 A38 L41 A39 | L42 A40 L43 A41 | L44 A42 L45 A43 | L46 A44 L47 A45 | L48 A46 L49 A47 | L50 A48 L51 A49 | L52 A50 L53 A51 | L54 A52 L55 A53 | L56 A54 L57 A55 | L58 A56 L59 A57 | L60 A58 L61 A59 | L62 A60 L63 A61 | L64 A62 L65 A63 | L66 A64 L67 A65 | L68 A66 L69 A67 | L70 A68 L71 A69 | L72 A70 L73 A71 | L74 A72 L75 A73 | L76 A74 L77 A75 | L78 A76 L79 A77 | L80 A78 L81 A79 | L82 A80 L83 A81 | L84 A82 L85 A83 | L86 A84 L87 A85 | L88 A86 L89 A87 | L90 A88 L91 A89 | L92 A90 L93 A91 | L94 A92 L95 A93 | L96 A94 L97 A95 | L98 A96 L99 A97 | L100 A98 L101 A99 | L102 A100 L103 A101 | L104 A102 L105 A103 | L106 A104 L107 A105 | L108 A106 L109 A107 | L110 A108 L111 A109 | L112 A110 L113 A111 | L114 A112 L115 A113 | L116 A114 L117 A115 | L118 A116 L119 A117 | L120 A118 L121 A119 | L122 A120 L123 A121 | L124 A122 L125 A123 | L126 A124 L127 A125 | L128 A126 L129 A127 | L130 A128 L131 A129 | L132 A130 L133 A131 | L134 A132 L135 A133 | L136 A134 L137 A135 | L138 A136 L139 A137 | L140 A138 L141 A139 | L142 A140 L143 A141 | L144 A142 L145 A143 | L146 A144 L147 A145 | L148 A146 L149 A147 | L150 A148 L151 A149 | L152 A150 L153 A151 | L154 A152 L155 A153 | L156 A154 L157 A155 | L158 A156 L159 A157 | L160 A158 L161 A159 | L0 L1 L4 A2 A3 | L0 L1 L3 A2 A3 in component "Wheel-Hub"
component "Wheel-Hub" placed x (1, 0, 0) y (0, 1, 0) z (0, 0, 1) at (0, 0, 0)
